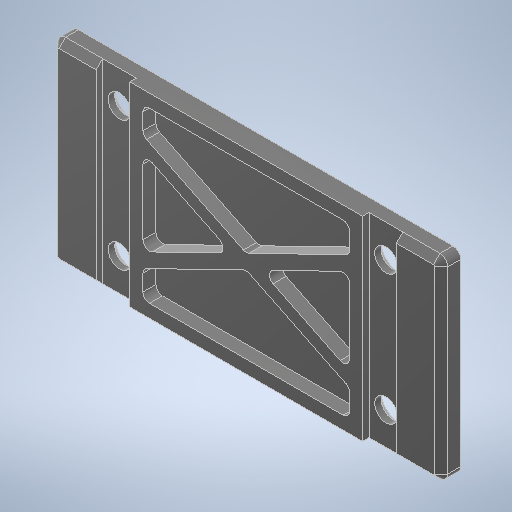
# Autodesk Inventor part: 3D_club
Saved by Autodesk Inventor 2025 (Build 290162000, 162)
## iProperties
Created: 2024-07-26
Part Number: 3D_club
Material: 一般
Document SubType Name: Modeling
Designer: 8326d
Density: 1 g/cm^3
Appearance: 滑らか - 黒
Author: 8326d
## iProperties of the stored document 3D_club_3D プリント.ipt
Created: 2024-08-04
Part Number: 3D_club_3D プリント
Material: 一般
Document SubType Name: Modeling
Designer: 8326d
Density: 1 g/cm^3
Appearance: 既定
Author: 8326d
Autodesk Inventor part; units mm, degrees
ref_plane "YZ Plane" through (0, 0, 0) normal (1, 0, 0) x (0, 1, 0)
ref_plane "XZ Plane" through (0, 0, 0) normal (0, 1, 0) x (-1, 0, 0)
ref_plane "XY Plane" through (0, 0, 0) normal (0, 0, 1) x (1, 0, 0)
sketch "スケッチ1" plane through (0, 0, 0) normal (0, 0, 1) x (1, 0, 0)
  line L0 (-30, -15) -> (30, -15)
  line L1 (30, -15) -> (30, 15)
  line L2 (30, 15) -> (-30, 15)
  line L3 (-30, 15) -> (-30, -15)
  line L4 (-30, -15) -> (30, 15) construction
  line L5 (30, -15) -> (-30, 15) construction
  point P0 (0, 0)
  dimension "d0" = 60
  dimension "d1" = 30
  constraints: 12 end point, 2 midpoint, 2 parallel, 1 horizontal, 1 perpendicular
  measures "d0" distance of L2.end L1.end
  measures "d1" distance of L1.end L0.end
extrude "押し出し1" add sketch "スケッチ1" along normal blind 3
sketch "スケッチ2" plane through (0, 0, 3) normal (0, 0, 1) x (1, 0, 0)
  line L0 (30, 15) -> (-30, 15) projected
  line L1 (-30, -15) -> (30, -15) projected
  line L2 (-17.9, 15) -> (-23.1, 15)
  line L3 (-23.1, 15) -> (-23.1, -15)
  line L4 (-23.1, -15) -> (-17.9, -15)
  line L5 (-17.9, -15) -> (-17.9, 15)
  line L6 (17.9, -15) -> (23.1, -15)
  line L7 (23.1, -15) -> (23.1, 15)
  line L8 (23.1, 15) -> (17.9, 15)
  line L9 (17.9, 15) -> (17.9, -15)
  point P0 (0, 0)
  dimension "d4" = 5.2
  dimension "d5" = 5.2
  dimension "d6" = 17.9
  dimension "d7" = 17.9
  constraints: 16 end point, 4 parallel, 4 point on line, 2 horizontal, 2 perpendicular
  measures "d4" distance between parallel lines of L3 L5
  measures "d5" distance between parallel lines of L7 L9
  measures "d6" distance from line of point (0, 0) L5
  measures "d7" distance from line of L9 point (0, 0)
extrude "押し出し2" cut sketch "スケッチ2" against normal blind 1 contours L7 L1 L9 L0 | L5 L1 L3 L0
sketch "スケッチ3" plane through (0, 0, 2) normal (0, 0, 1) x (1, 0, 0)
  line L0 (-23.1, 15) -> (-17.9, 15) projected
  line L1 (-17.9, -15) -> (-23.1, -15) projected
  line L2 (23.1, -15) -> (17.9, -15) projected
  line L3 (17.9, 15) -> (23.1, 15) projected
  line L4 (-20.5, 15) -> (-20.5, -15) construction
  line L5 (20.5, -15) -> (20.5, 15) construction
  point P0 (0, 0)
  point P1 (-20.5, 10)
  point P2 (-20.5, -10)
  point P3 (20.5, -10)
  point P4 (20.5, 10)
  dimension "d10" = 5
  dimension "d11" = 5
  dimension "d12" = 5
  dimension "d13" = 5
  constraints: 4 end point, 4 midpoint, 4 point on line
  measures "d10" distance from line of L0 point (-20.5, 10)
  measures "d11" distance from line of L1 point (-20.5, -10)
  measures "d12" distance from line of L3 point (20.5, 10)
  measures "d13" distance from line of L2 point (20.5, -10)
hole "穴1" at (-20.5, 10, 2) at (-20.5, -10, 2) at (20.5, -10, 2) at (20.5, 10, 2) direction (0, 0, -1) diameter 3.5 end through all
chamfer "面取り1" distance 1 angle 45 4 edges at (-20.5, -8.25, 0) (20.5, -8.25, 0) (-20.5, 11.75, 0) (20.5, 11.75, 0)
sketch "スケッチ4" plane through (0, 0, 3) normal (0, 0, 1) x (1, 0, 0)
  line L0 (17.9, -15) -> (17.9, 15) projected
  line L1 (17.9, 15) -> (-17.9, 15) projected
  line L2 (-17.9, 15) -> (-17.9, -15) projected
  line L3 (-17.9, -15) -> (17.9, -15) projected
  line L4 (-15.9, 13) -> (15.9, 13)
  line L5 (15.9, 13) -> (15.9, -13)
  line L6 (15.9, -13) -> (-15.9, -13)
  line L7 (-15.9, -13) -> (-15.9, 13)
  circle A0 centre (-20.5, 10) radius 1.75 projected
  circle A1 centre (20.5, -10) radius 1.75 projected
  circle A2 centre (20.5, 10) radius 1.75 projected
  circle A3 centre (-20.5, -10) radius 1.75 projected
  circle A4 centre (20.5, -10) radius 2.75 construction
  line L8 (-20.5, 10) -> (20.5, -10) construction
  line L9 (-20.5, -10) -> (20.5, 10) construction
  line L10 (-20.0616, -10.8988) -> (20.9384, 9.1012)
  line L11 (20.9384, 9.1012) -> (20.0616, 10.8988)
  line L12 (20.0616, 10.8988) -> (-20.9384, -9.1012)
  line L13 (-20.9384, -9.1012) -> (-20.0616, -10.8988)
  line L14 (-20.0616, -10.8988) -> (20.0616, 10.8988) construction
  line L15 (20.9384, 9.1012) -> (-20.9384, -9.1012) construction
  line L16 (20.0616, -10.8988) -> (-20.9384, 9.1012)
  line L17 (-20.9384, 9.1012) -> (-20.0616, 10.8988)
  line L18 (-20.0616, 10.8988) -> (20.9384, -9.1012)
  line L19 (20.9384, -9.1012) -> (20.0616, -10.8988)
  line L20 (20.0616, -10.8988) -> (-20.0616, 10.8988) construction
  line L21 (-20.9384, 9.1012) -> (20.9384, -9.1012) construction
  point P0 (0, 0)
  point P1 (15.9, -8.8687)
  point P2 (0, -1.1126)
  point P3 (-15.9, -8.8687)
  point P4 (2.2809, 0)
  point P5 (15.9, -6.6435)
  point P6 (15.9, 6.6435)
  point P7 (-2.2809, 0)
  point P8 (-15.9, 6.6435)
  point P9 (-15.9, -6.6435)
  point P10 (-15.9, 8.8687)
  point P11 (0, 1.1126)
  point P12 (15.9, 8.8687)
  dimension "d24" = 2
  dimension "d25" = 2
  dimension "d26" = 2
  constraints: 36 end point, 5 midpoint, 5 parallel, 2 perpendicular, 3 other
  measures "d24" distance between parallel lines of L1 L4
  measures "d25" distance of L11.end L10.end
  measures "d26" distance of L16.end L17.end
extrude "押し出し3" cut sketch "スケッチ4" against normal blind 2 contours L5 L6 L7 L10 L16 | L18 L10 L5 | L12 L7 L16 | L12 L18 L7 L4 L5
fillet "フィレット1" radius 1 16 edges at (-15.9, 6.6435, 2) (-15.9, -6.6435, 2) (-2.2809, 0, 2) (0, -1.1126, 2) (2.2809, 0, 2) (15.9, -6.6435, 2) (15.9, -8.8687, 2) (15.9, -13, 2) (-15.9, -13, 2) (-15.9, -8.8687, 2) (15.9, 6.6435, 2) (15.9, 8.8687, 2) (15.9, 13, 2) (-15.9, 13, 2) (-15.9, 8.8687, 2) (0, 1.1126, 2)
fillet "フィレット2" radius 1.2 4 edges at (-30, 15, 1.5) (-30, -15, 1.5) (30, -15, 1.5) (30, 15, 1.5)
chamfer "面取り2" distance 1 angle 45 10 edges at (-30, 0, 3) (-29.6485, -14.6485, 3) (-25.95, -15, 3) (-29.6485, 14.6485, 3) (-25.95, 15, 3) (30, 0, 3) (29.6485, 14.6485, 3) (25.95, 15, 3) (29.6485, -14.6485, 3) (25.95, -15, 3)
equation "\"d5\" = d4"
equation "\"d7\" = d6"
equation "\"d11\" = d10"
equation "\"d12\" = d10"
equation "\"d13\" = d10"
